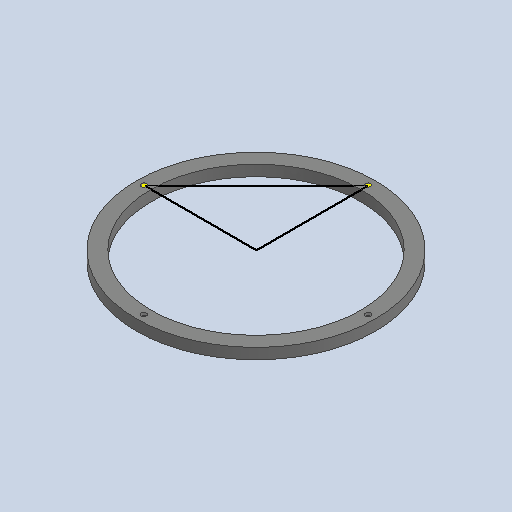
# Autodesk Inventor part: InnerBearingTable
Saved by Autodesk Inventor 2023 (Build 270158000, 158)
## iProperties
Created: 2023-03-23
Part Number: InnerBearingTable
Material: Generic
Document SubType Name: Modeling
Designer: czapa
Density: 1 g/cm^3
Appearance: Default
Author: czapa
Autodesk Inventor part; units mm, degrees
ref_plane "YZ Plane" through (0, 0, 0) normal (1, 0, 0) x (0, 1, 0)
ref_plane "XZ Plane" through (0, 0, 0) normal (0, 1, 0) x (-1, 0, 0)
ref_plane "XY Plane" through (0, 0, 0) normal (0, 0, 1) x (1, 0, 0)
sketch "Sketch1" plane through (0, 0, 0) normal (0, 1, 0) x (-1, 0, 0)
  circle A0 centre (0, 0) radius 97.5
  circle A1 centre (0, 0) radius 111.25
  dimension "d0" = 195
  dimension "d1" = 222.5
  constraints: 2 centre point, 2 coincident
  measures "d0" diameter of A0
  measures "d1" diameter of A1
extrude "Extrusion1" add sketch "Sketch1" along normal blind 10
sketch "Sketch2" plane through (0, 10, 0) normal (0, 1, 0) x (1, 0, 0)
  line L0 (0, 0) -> (0, 104.375)
  dimension "d4" = 104.375
  constraints: 2 end point, 1 coincident, 1 vertical
  measures "d4" distance of L0.start L0.end
hole "Hole1" at (0, 10, -104.375) direction (0, -1, 0) diameter 2.5 end through all countersink diameter 5 countersink angle 90
pattern_circular "Circular Pattern1" count 4 over 360 about axis through (0, -10, 0) along (0, 1, 0) of "Hole1"
sketch "Sketch3" plane through (0, 10, 0) normal (0, 1, 0) x (1, 0, 0)
  circle A0 centre (-104.375, 0) radius 1.25 projected
  line L0 (-104.375, 0) -> (0, 0)
  circle A1 centre (0, 104.375) radius 1.25 projected
  line L1 (0, 0) -> (0, 104.375)
  line L2 (0, 104.375) -> (-104.375, 0)
  constraints: 6 end point, 1 horizontal, 1 perpendicular
body "Solid1"
